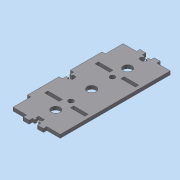
# Autodesk Inventor part: X-Anchor_Front-Outer
Saved by Autodesk Inventor 2016 SP1 (Build 200210100, 210)
## iProperties
Created: 2016-02-24
Part Number: X-Anchor_Front-Outer
Material: Generic
Document SubType Name: Modeling
Designer: Mohamed A.
Density: 1 g/cm^3
Appearance: Default
Author: Mohamed A.
Autodesk Inventor part; units mm, degrees
ref_plane "YZ Plane" through (0, 0, 0) normal (1, 0, 0) x (0, 1, 0)
ref_plane "XZ Plane" through (0, 0, 0) normal (0, 1, 0) x (-1, 0, 0)
ref_plane "XY Plane" through (0, 0, 0) normal (0, 0, 1) x (1, 0, 0)
sketch "Sketch2" plane through (0, 0, 0) normal (0, 0, 1) x (1, 0, 0)
  circle A0 centre (0, 0) radius 11 construction
  circle A1 centre (0, 32) radius 3.9 projected
  circle A2 centre (0, -32) radius 3.9 projected
  circle A3 centre (15.5, -15.5) radius 1.4 projected
  circle A4 centre (-15.5, -15.5) radius 1.4 projected
  circle A5 centre (-15.5, 15.5) radius 1.4 projected
  circle A6 centre (15.5, 15.5) radius 1.4 projected
  line L0 (-2.65, 44.6) -> (-1.5, 44.6) projected
  line L1 (-1.5, 44.6) -> (-1.5, 44) projected
  line L2 (-1.5, 44) -> (1.5, 44) projected
  line L3 (1.5, 44) -> (1.5, 44.6) projected
  line L4 (1.5, 44.6) -> (2.65, 44.6) projected
  line L5 (2.65, 44.6) -> (2.65, 47) projected
  line L6 (2.65, 47) -> (1.5, 47) projected
  line L7 (1.5, 47) -> (1.5, 49) projected
  line L8 (1.5, 49) -> (3.75, 49) projected
  line L9 (3.75, 49) -> (3.75, 52) projected
  line L10 (3.75, 52) -> (9, 52) projected
  line L11 (9, 52) -> (9, 49) projected
  line L12 (9, 49) -> (21, 49) projected
  line L13 (21, 49) -> (21, -49) projected
  line L14 (21, -49) -> (9, -49) projected
  line L15 (9, -49) -> (9, -52) projected
  line L16 (9, -52) -> (3.75, -52) projected
  line L17 (3.75, -52) -> (3.75, -49) projected
  line L18 (3.75, -49) -> (1.5, -49) projected
  line L19 (1.5, -49) -> (1.5, -47) projected
  line L20 (1.5, -47) -> (2.65, -47) projected
  line L21 (2.65, -47) -> (2.65, -44.6) projected
  line L22 (2.65, -44.6) -> (-2.65, -44.6) projected
  line L23 (-2.65, -44.6) -> (-2.65, -47) projected
  line L24 (-2.65, -47) -> (-1.5, -47) projected
  line L25 (-1.5, -47) -> (-1.5, -49) projected
  line L26 (-1.5, -49) -> (-3.75, -49) projected
  line L27 (-3.75, -49) -> (-3.75, -52) projected
  line L28 (-3.75, -52) -> (-9, -52) projected
  line L29 (-9, -52) -> (-9, -49) projected
  line L30 (-9, -49) -> (-21, -49) projected
  line L31 (-21, -49) -> (-21, -33.1667) projected
  line L32 (-21, -33.1667) -> (-24, -33.1667) projected
  line L33 (-24, -33.1667) -> (-24, -5) projected
  line L34 (-24, -5) -> (-21, -5) projected
  line L35 (-21, -5) -> (-21, -1.5) projected
  line L36 (-21, -1.5) -> (-19, -1.5) projected
  line L37 (-19, -1.5) -> (-19, -2.65) projected
  line L38 (-19, -2.65) -> (-16.6, -2.65) projected
  line L39 (-16.6, -2.65) -> (-16.6, -1.5) projected
  line L40 (-16.6, -1.5) -> (-16, -1.5) projected
  line L41 (-16, -1.5) -> (-16, 1.5) projected
  line L42 (-16, 1.5) -> (-16.6, 1.5) projected
  line L43 (-16.6, 1.5) -> (-16.6, 2.65) projected
  line L44 (-16.6, 2.65) -> (-19, 2.65) projected
  line L45 (-19, 2.65) -> (-19, 1.5) projected
  line L46 (-19, 1.5) -> (-21, 1.5) projected
  line L47 (-21, 1.5) -> (-21, 5) projected
  line L48 (-21, 5) -> (-24, 5) projected
  line L49 (-24, 5) -> (-24, 33.1667) projected
  line L50 (-24, 33.1667) -> (-21, 33.1667) projected
  line L51 (-21, 33.1667) -> (-21, 49) projected
  line L52 (-21, 49) -> (-9, 49) projected
  line L53 (-9, 49) -> (-9, 52) projected
  line L54 (-9, 52) -> (-3.75, 52) projected
  line L55 (-3.75, 52) -> (-3.75, 49) projected
  line L56 (-3.75, 49) -> (-1.5, 49) projected
  line L57 (-1.5, 49) -> (-1.5, 47) projected
  line L58 (-1.5, 47) -> (-2.65, 47) projected
  line L59 (-2.65, 47) -> (-2.65, 44.6) projected
  circle A7 centre (0, 0) radius 4
  line L60 (-5, -21) -> (-18, -21) projected
  line L61 (-18, -21) -> (-18, -24) projected
  line L62 (-18, -24) -> (-5, -24) projected
  line L63 (-5, -24) -> (-5, -21) projected
  line L64 (5, -24) -> (18, -24) projected
  line L65 (18, -24) -> (18, -21) projected
  line L66 (18, -21) -> (5, -21) projected
  line L67 (5, -21) -> (5, -24) projected
  line L68 (-5, 24) -> (-18, 24) projected
  line L69 (-18, 24) -> (-18, 21) projected
  line L70 (-18, 21) -> (-5, 21) projected
  line L71 (-5, 21) -> (-5, 24) projected
  line L72 (5, 21) -> (18, 21) projected
  line L73 (18, 21) -> (18, 24) projected
  line L74 (18, 24) -> (5, 24) projected
  line L75 (5, 24) -> (5, 21) projected
  circle A8 centre (0, -18.5) radius 2.4 construction
  circle A9 centre (0, 18.5) radius 2.4 construction
  circle A10 centre (0, 18.5) radius 2.2
  circle A11 centre (0, -18.5) radius 2.2
  dimension "d6" = 8
  dimension "d9" = 0.2
  dimension "d10" = 0.2
  constraints: 3 centre point, 1 coincident
  measures "d6" diameter of A7
  measures "d9" radial gap between concentric circles of A9 A10
  measures "d10" radial gap between concentric circles of A8 A11
extrude "Extrusion1" add sketch "Sketch2" along normal blind 3 contours A3 | A4 | A5 | A6 | L0 L1 L2 L3 L4 L5 L6 L7 L8 L9 L10 L11 L12 L13 L14 L15 L16 L17 L18 L19 L20 L21 L22 L23 L24 L25 L26 L27 L28 L29 L30 L31 L32 L33 L34 L35 L36 L37 L38 L39 L40 L41 L42 L43 L44 L45 L46 L47 L48 L49 L50 L51 L52 L53 L54 L55 L56 L57 L58 L59
body "Solid1"
